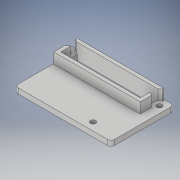
# Autodesk Inventor part: MidPlate v2
Saved by Autodesk Inventor 2019 (Build 230136000, 136)
## iProperties
Created: 2019-02-19
Part Number: MidPlate v2
Material: Generic
Document SubType Name: Modeling
Designer: Jared
Density: 1 g/cm^3
Appearance: Default
Author: Jared
Autodesk Inventor part; units mm, degrees
ref_plane "YZ Plane" through (0, 0, 0) normal (1, 0, 0) x (0, 1, 0)
ref_plane "XZ Plane" through (0, 0, 0) normal (0, 1, 0) x (-1, 0, 0)
ref_plane "XY Plane" through (0, 0, 0) normal (0, 0, 1) x (1, 0, 0)
sketch "Sketch1" plane through (0, 0, 0) normal (0, 1, 0) x (-1, 0, 0)
  line L0 (2, 0) -> (53, 0)
  line L1 (58, -36) -> (2, -36)
  line L2 (0, -34) -> (0, -2)
  line L3 (60, -34) -> (60, -29)
  line L4 (58, -27) -> (55, -27)
  line L5 (55, -27) -> (55, -2)
  arc A0 (58, -36) -> (60, -34) centre (58, -34) ccw
  arc A1 (0, -34) -> (2, -36) centre (2, -34) ccw
  arc A2 (55, -2) -> (53, 0) centre (53, -2) ccw
  arc A3 (2, 0) -> (0, -2) centre (2, -2) ccw
  arc A4 (60, -29) -> (58, -27) centre (58, -29) ccw
  point P0 (0, 0)
  point P1 (60, -36)
  point P2 (55, 0)
  point P3 (0, -36)
  point P4 (60, -27)
  dimension "d0" = 60
  dimension "d47" = 36
  dimension "d48" = 9
  dimension "d49" = 5
  dimension "d68" = 2
  dimension "d87" = 2
  constraints: 12 end point, 10 point on circle, 10 point on line, 10 tangent, 5 centre point, 3 equal radius, 3 perpendicular, 1 horizontal, 1 parallel, 1 vertical
  measures "d0" distance of point (60, -36) point (0, -36)
  measures "d47" distance of point (0, -36) point (0, 0)
  measures "d48" distance of point (60, -36) point (60, -27)
  measures "d49" distance of point (60, -27) L4.end
  measures "d68" radius of A0
  measures "d87" radius of A4
extrude "Extrusion1" add sketch "Sketch1" along normal blind 3
sketch "Sketch7" plane through (0, 3, 0) normal (0, 1, 0) x (1, 0, 0)
  line L0 (-53, 0) -> (-2, 0) projected
  line L1 (0, 2) -> (0, 34) projected
  line L2 (-2, 36) -> (-58, 36) projected
  line L3 (-56.25, 31.5) -> (-3.75, 31.5)
  line L4 (-3.75, 31.5) -> (-3.75, 4.5)
  line L5 (-3.75, 4.5) -> (-56.25, 4.5)
  line L6 (-56.25, 4.5) -> (-56.25, 31.5)
  line L7 (-55, 27) -> (-55, 2) projected
  line L8 (-60, 34) -> (-60, 29) projected
  line L9 (-58, 27) -> (-55, 27) projected
  arc A0 (-55, 2) -> (-53, 0) centre (-53, 2) ccw projected
  arc A1 (-2, 0) -> (0, 2) centre (-2, 2) ccw projected
  arc A2 (0, 34) -> (-2, 36) centre (-2, 34) ccw projected
  arc A3 (-58, 36) -> (-60, 34) centre (-58, 34) ccw projected
  arc A4 (-60, 29) -> (-58, 27) centre (-58, 29) ccw projected
  point P0 (-14.75, 4.5)
  dimension "d42" = 27
  dimension "d43" = 52.5
  dimension "d44" = 4.5
  dimension "d45" = 11
  dimension "d50" = 3.75
  constraints: 8 end point, 2 parallel, 1 horizontal, 1 perpendicular, 1 point on line
  measures "d42" distance of L5.end L3.start
  measures "d43" distance of L3.start L3.end
  measures "d44" distance between parallel lines of L2 L3
  measures "d45" distance from line of L4 point (-14.75, 4.5)
  measures "d50" distance between parallel lines of L8 L6
hole "Hole1" at (-56.25, 3, -31.5) at (-3.75, 3, -31.5) at (-14.75, 3, -4.5) direction (0, -1, 0) diameter 3 depth 10.25
sketch "Sketch8" plane through (0, 3, 0) normal (0, 1, 0) x (1, 0, 0)
  line L0 (-52.75, 33.5) -> (-7.25, 33.5)
  line L1 (-7.25, 24) -> (-52.75, 24)
  circle A0 centre (-56.25, 31.5) radius 1.5 projected
  circle A1 centre (-3.75, 31.5) radius 1.5 projected
  circle A2 centre (-56.25, 31.5) radius 3.5
  circle A3 centre (-3.75, 31.5) radius 3.5
  line L2 (-2, 36) -> (-58, 36) projected
  line L3 (-54.75, 28.3377) -> (-54.75, 22)
  line L4 (-54.75, 22) -> (-5.25, 22)
  line L5 (-5.25, 35.5) -> (-54.75, 35.5)
  line L6 (-54.75, 35.5) -> (-54.75, 34.6623)
  line L7 (-52.75, 33.5) -> (-53.3777, 33.5)
  line L8 (-52.75, 24) -> (-52.75, 29.5)
  line L9 (-52.75, 29.5) -> (-52.75, 31.5)
  line L10 (-52.75, 33.5) -> (-52.75, 31.5)
  line L11 (-52.75, 29.5) -> (-53.3777, 29.5)
  line L12 (-7.25, 33.5) -> (-7.25, 31.5)
  line L13 (-7.25, 31.5) -> (-7.25, 29.5)
  line L14 (-7.25, 29.5) -> (-7.25, 24)
  line L15 (-7.25, 33.5) -> (-6.6223, 33.5)
  line L16 (-7.25, 29.5) -> (-6.6223, 29.5)
  line L17 (-5.25, 35.5) -> (-5.25, 34.6623)
  line L18 (-5.25, 28.3377) -> (-5.25, 22)
  point P0 (0, 0)
  dimension "d73" = 9.5
  dimension "d74" = 45.5
  dimension "d75" = 7
  dimension "d76" = 7
  dimension "d77" = 2.5
  dimension "d78" = 2
  dimension "d81" = 2
  dimension "d82" = 9.5
  dimension "d83" = 2
  dimension "d85" = 49.5
  dimension "d86" = 49.5
  constraints: 36 end point, 10 point on circle, 4 point on line, 4 vertical, 3 collinear, 3 tangent, 2 centre point, 2 concentric, 2 horizontal, 2 parallel, 2 perpendicular
  measures "d73" distance of L1.end L0.start
  measures "d74" distance of L1.start L1.end
  measures "d75" diameter of A2
  measures "d76" diameter of A3
  measures "d77" distance between parallel lines of L2 L0
  measures "d78" distance between parallel lines of L1 L4
  measures "d81" distance between parallel lines of L0 L5
  measures "d82" distance between parallel lines of L0 L1
  measures "d83" distance between parallel lines of L8 L3
  measures "d85" distance between parallel lines of L3 L18
  measures "d86" distance between parallel lines of L3 L17
extrude "Extrusion6" add sketch "Sketch8" along normal blind 6 contours L7 A2 L6 L5 L17 A3 L15 L0 | L11 L8 L1 L14 L16 A3 L18 L4 L3 A2
sketch "Sketch9" plane through (0, 3, 0) normal (0, 1, 0) x (1, 0, 0)
  line L0 (-52.75, 29.5) -> (-52.75, 24) projected
  line L1 (-52.75, 24) -> (-7.25, 24) projected
  line L2 (-7.25, 24) -> (-7.25, 29.5) projected
  line L3 (-6.6223, 33.5) -> (-53.3777, 33.5) projected
  line L4 (-52.75, 29.5) -> (-52.75, 33.5)
  line L5 (-7.25, 29.5) -> (-6.6223, 29.5) projected
  line L6 (-7.25, 29.5) -> (-7.25, 33.5)
  point P0 (0, 0)
  constraints: 4 end point, 2 point on line, 1 perpendicular, 1 vertical
extrude "Extrusion7" cut sketch "Sketch9" against normal up to next
body "Solid1"
